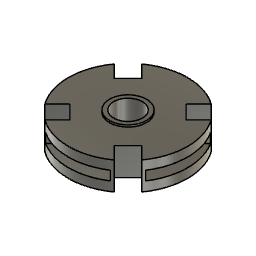
Piston Internal Gear (Autodesk Fusion 360 design; units mm, degrees)
Autodesk Fusion 360 part; units mm, degrees
sketch "Sketch1" plane through (0, 0, 0) normal (0, 0, 1) x (1, 0, 0) in component "Component"
  circle A0 centre (0, 0) radius 1.55
  circle A1 centre (0, 0) radius 6.45
  line L0 (-3.8891, 2.4042) -> (-5.2425, 3.7575)
  line L1 (-3.1466, 3.1466) -> (-3.8891, 2.4042)
  line L2 (-3.1466, 3.1466) -> (-2.4042, 3.8891)
  line L3 (-2.4042, 3.8891) -> (-3.7575, 5.2425)
  line L4 (-2.4042, -3.8891) -> (-3.7575, -5.2425)
  line L5 (-3.1466, -3.1466) -> (-2.4042, -3.8891)
  line L6 (-3.1466, -3.1466) -> (-3.8891, -2.4042)
  line L7 (-3.8891, -2.4042) -> (-5.2425, -3.7575)
  line L8 (3.8891, -2.4042) -> (5.2425, -3.7575)
  line L9 (3.1466, -3.1466) -> (3.8891, -2.4042)
  line L10 (3.1466, -3.1466) -> (2.4042, -3.8891)
  line L11 (2.4042, -3.8891) -> (3.7575, -5.2425)
  line L12 (2.4042, 3.8891) -> (3.7575, 5.2425)
  line L13 (3.1466, 3.1466) -> (2.4042, 3.8891)
  line L14 (3.1466, 3.1466) -> (3.8891, 2.4042)
  line L15 (3.8891, 2.4042) -> (5.2425, 3.7575)
  circle A2 centre (0, 0) radius 2
  line L16 (-1.9799, 3.8891) -> (-3.5052, 5.4144)
  line L17 (-2.9345, 2.9345) -> (-1.9799, 3.8891)
  line L18 (-2.9345, 2.9345) -> (-3.8891, 1.9799)
  line L19 (-3.8891, 1.9799) -> (-5.4144, 3.5052)
  line L20 (-3.8891, -1.9799) -> (-5.4144, -3.5052)
  line L21 (-2.9345, -2.9345) -> (-3.8891, -1.9799)
  line L22 (-2.9345, -2.9345) -> (-1.9799, -3.8891)
  line L23 (-1.9799, -3.8891) -> (-3.5052, -5.4144)
  line L24 (1.9799, -3.8891) -> (3.5052, -5.4144)
  line L25 (2.9345, -2.9345) -> (1.9799, -3.8891)
  line L26 (2.9345, -2.9345) -> (3.8891, -1.9799)
  line L27 (3.8891, -1.9799) -> (5.4144, -3.5052)
  line L28 (3.8891, 1.9799) -> (5.4144, 3.5052)
  line L29 (2.9345, 2.9345) -> (3.8891, 1.9799)
  line L30 (2.9345, 2.9345) -> (1.9799, 3.8891)
  line L31 (1.9799, 3.8891) -> (3.5052, 5.4144)
  dimension "d1" = 3.1
  dimension "d2" = 12.9
  dimension "d13" = 360
  constraint coincident A0.centre A1.centre
  constraint concentric A0 A1
  constraint parallel L3 L16
  constraint parallel L2 L17
  constraint parallel L1 L18
  constraint parallel L0 L19
  constraint coincident A1 L16.end
  constraint coincident A1 L19.end
  measures "d1" diameter of A0
  measures "d2" diameter of A1
extrude "Extrude1" add sketch "Sketch1" along normal blind 3 contours A1 L16 L17 L18 L19 L20 L21 L22 L23 L24 L25 L26 L27 L28 L29 L30 L31 | A1 L12 L13 L14 L15 L28 L29 L30 L31 | A1 L8 L9 L10 L11 L24 L25 L26 L27 | A1 L0 L1 L2 L3 L16 L17 L18 L19 | A1 L4 L5 L6 L7 L20 L21 L22 L23 | A2 in component "Component"
extrude "Extrude2" cut 1 faces at (0, 4.7427, 0) along direction (0, 0, 1) blind 2 in component "Component"
extrude "Extrude3" add sketch "Sketch1" along normal blind 2 contours A1 L12 L13 L14 L15 L28 L29 L30 L31 | A1 L8 L9 L10 L11 L24 L25 L26 L27 | A1 L0 L1 L2 L3 L16 L17 L18 L19 | A1 L4 L5 L6 L7 L20 L21 L22 L23 | A2 in component "Component"
extrude "Extrude4" add sketch "Sketch1" along normal blind 1 contours A1 L16 L17 L18 L19 L20 L21 L22 L23 L24 L25 L26 L27 L28 L29 L30 L31 in component "Component"
extrude "Extrude5" cut sketch "Sketch1" along normal blind 5 contours A2 in component "Component"
extrude "Extrude6" add sketch "Sketch1" along normal blind 3.2 contours A2 in component "Component"
extrude "Extrude7" add sketch "Sketch1" against normal blind 0.2 contours A2 in component "Component"
component "Component" placed x (1, 0, 0) y (0, 1, 0) z (0, 0, 1) at (0, 0, 0)
